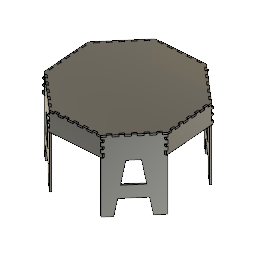
table v11 (Autodesk Fusion 360 design; units mm, degrees)
Autodesk Fusion 360 part; units mm, degrees
note: some values were not read from the file. Chosen so that the rebuilt part matches the saved one: a direction. Set by a fixed rule: which face or edge a step refers to.
sketch "TableTopSide Sketch" plane through (0, 0, 0) normal (0, 0, 1) x (1, 0, 0)
  line L0 (0, 0) -> (123.0551, 378.7517)
  line L1 (123.0551, 378.7517) -> (354.831, 180.8048)
  line L2 (354.831, 180.8048) -> (0, 0)
  dimension "d1" = 45
  dimension "d18" = 304.8
  measures "d1" angle of L0 L2
extrude "Extrude1" add sketch "TableTopSide Sketch" along normal blind 11 makes body 1
sketch "TableTopSideFinger Sketch" plane through (238.9431, 279.7782, 0) normal (0.649432, 0.76042, 0) x (-0.76042, 0.649432, 0)
  line L0 (-152.4, 0) -> (152.4, 0)
  line L1 (152.4, 0) -> (152.4, 11)
  line L2 (152.4, 11) -> (-152.4, 11)
  line L3 (-152.4, 11) -> (-152.4, 0)
  line L4 (-127, 11) -> (-101.6, 11)
  line L5 (-101.6, 11) -> (-101.6, 0)
  line L6 (-101.6, 0) -> (-127, 0)
  line L7 (-127, 0) -> (-127, 11)
  dimension "d23" = 25.4
  dimension "d24" = 25.4
  measures "d23" distance of L3 L7
  measures "d24" distance of L5 L7
extrude "Extrude3" cut sketch "TableTopSideFinger Sketch" against normal blind 11 contours L0 L2 L4 L5 L6 L7 bodies 1
pattern_linear "R-Pattern2" count 5 spacing 57.15 along (-0.76042, 0.649432, 0) of "Extrude3"
pattern_circular "C-Pattern1" count 8 over 360 about axis through (0, 0, 1.75) along (0, 0, 1) of bodies 1 makes body 2 at (-37.6656, 235.7218, 11) makes body 3 at (-193.3141, 140.0469, 11) makes body 4 at (-235.7218, -37.6656, 11) makes body 5 at (-169.0189, -168.5707, 11) makes body 6 at (37.6656, -235.7218, 11) makes body 7 at (193.3141, -140.0469, 11) makes body 8 at (235.7218, 37.6656, 11)
sketch "Leg Sketch" plane through (238.9431, 279.7782, 0) normal (0.649432, 0.76042, 0) x (-0.76042, 0.649432, 0)
  line L0 (-152.4, 11) -> (152.4, 11)
  line L1 (152.4, 11) -> (152.4, -441.7199)
  line L2 (-152.4, -441.7199) -> (-152.4, 11)
  line L3 (152.4, 0) -> (152.4, 11)
  line L4 (-92.9491, -441.7199) -> (-38.655, -133.8025)
  line L5 (-38.655, -133.8025) -> (31.7592, -133.8025)
  line L6 (31.7592, -133.8025) -> (86.0534, -441.7199)
  line L7 (152.4, -441.7199) -> (86.0534, -441.7199)
  line L8 (-92.9491, -441.7199) -> (-152.4, -441.7199)
  line L9 (-75.5345, -342.9565) -> (68.6387, -342.9565)
  line L10 (-62.4641, -268.8305) -> (55.5683, -268.8305)
  dimension "d36" = 100
  dimension "d37" = 100
  measures "d36" angle of L4 L8
  measures "d37" angle of L6 L7
extrude "Extrude4" add sketch "Leg Sketch" against normal blind 11 separate body contours L0 L1 L2 L3 L4 L5 L6 L7 L8 | L4 L6 L9 L10 makes body 9
combine "Combine1" operation cut target body 9 tool bodies 1 keep tools
sketch "SideCover Sketch" plane through (-28.8748, 366.7914, 0) normal (-0.07848, 0.996916, 0) x (-0.996916, -0.07848, 0)
  line L0 (-127, 0) -> (-127, 11)
  line L1 (-127, 11) -> (-152.4, 11)
  line L2 (-152.4, 11) -> (-152.4, 0)
  line L3 (-152.4, 0) -> (-127, 0)
  line L4 (0, 11) -> (0, -115) construction
  line L5 (-163.4, 11) -> (163.4, 11)
  line L6 (163.4, 11) -> (163.4, -111.0995)
  line L7 (163.4, -111.0995) -> (-163.4, -111.0995)
  line L8 (-163.4, -111.0995) -> (-163.4, 11)
  line L9 (12.7, 11) -> (44.45, 11)
  line L10 (152.4, 11) -> (152.4, -33.5866) construction
  line L11 (-152.4, 11) -> (-152.4, -39.2984)
  dimension "d61" = 11
  dimension "d62" = 11
  measures "d61" distance of L8 L11
  measures "d62" distance of L6 L10
extrude "Extrude5" add sketch "SideCover Sketch" against normal blind 11 separate body makes body 10
sketch "SideCoverFinger Sketch" plane through (162.896, 12.8236, 0) normal (0.996916, 0.07848, 0) x (-0.07848, 0.996916, 0)
  line L0 (367.9261, -115) -> (367.9261, 0)
  line L1 (367.9261, 0) -> (355.9261, 0)
  line L2 (355.9261, 0) -> (355.9261, -115)
  line L3 (355.9261, -115) -> (367.9261, -115)
  line L4 (355.9261, -13.4) -> (367.9261, -13.4)
  line L5 (367.9261, -13.4) -> (367.9261, 12)
  line L6 (367.9261, 12) -> (355.9261, 12)
  line L7 (355.9261, 12) -> (355.9261, -13.4)
  line L8 (367.9261, 12) -> (152.4, 12)
  line L9 (367.9261, -111.0995) -> (367.9261, 11)
  line L10 (367.9261, 11) -> (356.9261, 11)
  line L11 (356.9261, 11) -> (356.9261, -111.0995)
  line L12 (356.9261, -111.0995) -> (367.9261, -111.0995)
  dimension "d46" = 25.4
  measures "d46" distance of L4 L6
extrude "Extrude6" cut sketch "SideCoverFinger Sketch" against normal blind 11 contours L0 L1 L4 L5 L9 L11 | L1 L2 L4 L7 L11 | L1 L5 L9 L10 L11 | L1 L5 L6 L7 L8 L10 L11 bodies 10
pattern_linear "R-Pattern3" count 3 spacing 38.1 along (0, 0, -1) of "Extrude6"
extrude "Extrude8" cut 3 faces at (123.3429, 375.0963, -5.2667) (123.6307, 371.441, -34.5667) (123.6307, 371.441, -72.6667) along direction (0.996916, 0.07848, 0) blind 12 start surface through (-191.7708, 353.9677, 11) normal (-0.996916, -0.07848, 0) on bodies 10 bodies 10
combine "Combine3" operation cut target body 9 tool bodies 10 keep tools
revolve "Revolve1" cut 1 faces at (126.0597, 367.9542, -103.933) angle 45 about axis through (134.8845, 368.6489, -64.2) along (0, 0, 1) on bodies 9 bodies 9
pattern_circular "C-Pattern3" count 4 over 360 about axis through (0, 0, 1.75) along (0, 0, 1) of bodies 10 makes body 11 at (-351.8908, -77.9902, -43.0333) makes body 12 at (77.9902, -351.8908, -43.0333) makes body 13 at (351.8908, 77.9902, -43.0333)
combine "Combine4" operation cut target body 9 tool bodies 13 keep tools
combine "Combine5" operation add target body 1 tool bodies 6 3 2 4 5 7 8 keep tools
revolve "Revolve2" cut 1 faces at (343.7225, 181.7504, -103.933) angle 45 about axis through (343.0017, 190.9076, -51.5) along (0, 0, -1) on bodies 9 bodies 9
pattern_circular "C-Pattern5" count 4 over 360 about axis through (0, 0, 1.75) along (0, 0, 1) of bodies 9 makes body 14 at (-360.6193, 144.2864, -298.592) makes body 15 at (-144.2864, -360.6193, -298.592) makes body 16 at (360.6193, -144.2864, -298.592)
sketch "Sketch8" plane through (366.7914, 28.8748, 0) normal (0.996916, 0.07848, 0) x (-0.07848, 0.996916, 0)
  line L0 (718.5635, -1934.0264) -> (737.8781, -1950.5219)
  line L1 (737.8781, -1950.5219) -> (745.0219, -1942.1573)
  line L2 (745.0219, -1942.1573) -> (764.3365, -1958.6529)
  line L3 (764.3365, -1958.6529) -> (757.1928, -1967.0175)
  line L4 (757.1928, -1967.0175) -> (781.3361, -1987.637)
  line L5 (781.3361, -1987.637) -> (788.4799, -1979.2724)
  line L6 (788.4799, -1979.2724) -> (807.7945, -1995.768)
  line L7 (807.7945, -1995.768) -> (800.6508, -2004.1326)
  line L8 (800.6508, -2004.1326) -> (824.7941, -2024.752)
  line L9 (824.7941, -2024.752) -> (831.9378, -2016.3874)
  line L10 (831.9378, -2016.3874) -> (851.2525, -2032.883)
  line L11 (851.2525, -2032.883) -> (844.1087, -2041.2476)
  line L12 (844.1087, -2041.2476) -> (868.2521, -2061.8671)
  line L13 (868.2521, -2061.8671) -> (875.3958, -2053.5025)
  line L14 (875.3958, -2053.5025) -> (894.7105, -2069.998)
  line L15 (894.7105, -2069.998) -> (887.5667, -2078.3627)
  line L16 (887.5667, -2078.3627) -> (911.71, -2098.9821)
  line L17 (911.71, -2098.9821) -> (918.8538, -2090.6175)
  line L18 (918.8538, -2090.6175) -> (938.1684, -2107.1131)
  line L19 (938.1684, -2107.1131) -> (931.0247, -2115.4777)
  line L20 (931.0247, -2115.4777) -> (950.3393, -2131.9733)
  line L21 (950.3393, -2131.9733) -> (975.661, -2129.9799)
  line L22 (975.661, -2129.9799) -> (974.7977, -2119.0138)
  line L23 (974.7977, -2119.0138) -> (1000.1194, -2117.0204)
  line L24 (1000.1194, -2117.0204) -> (1000.9827, -2127.9865)
  line L25 (1000.9827, -2127.9865) -> (1032.6347, -2125.4948)
  line L26 (1032.6347, -2125.4948) -> (1031.7715, -2114.5287)
  line L27 (1031.7715, -2114.5287) -> (1057.0931, -2112.5353)
  line L28 (1057.0931, -2112.5353) -> (1057.9564, -2123.5014)
  line L29 (1057.9564, -2123.5014) -> (1089.6085, -2121.0096)
  line L30 (1089.6085, -2121.0096) -> (1088.7452, -2110.0436)
  line L31 (1088.7452, -2110.0436) -> (1114.0668, -2108.0502)
  line L32 (1114.0668, -2108.0502) -> (1114.9301, -2119.0163)
  line L33 (1114.9301, -2119.0163) -> (1146.5822, -2116.5245)
  line L34 (1146.5822, -2116.5245) -> (1145.7189, -2105.5584)
  line L35 (1145.7189, -2105.5584) -> (1171.0406, -2103.5651)
  line L36 (1171.0406, -2103.5651) -> (1171.9039, -2114.5311)
  line L37 (1171.9039, -2114.5311) -> (1203.5559, -2112.0394)
  line L38 (1203.5559, -2112.0394) -> (1202.6926, -2101.0733)
  line L39 (1202.6926, -2101.0733) -> (1228.0143, -2099.0799)
  line L40 (1228.0143, -2099.0799) -> (1228.8776, -2110.046)
  line L41 (1228.8776, -2110.046) -> (1254.1992, -2108.0526)
  line L42 (1254.1992, -2108.0526) -> (1270.6948, -2088.738)
  line L43 (1270.6948, -2088.738) -> (1262.3302, -2081.5942)
  line L44 (1262.3302, -2081.5942) -> (1278.8258, -2062.2795)
  line L45 (1278.8258, -2062.2795) -> (1287.1904, -2069.4233)
  line L46 (1287.1904, -2069.4233) -> (1307.8099, -2045.28)
  line L47 (1307.8099, -2045.28) -> (1299.4453, -2038.1362)
  line L48 (1299.4453, -2038.1362) -> (1315.9408, -2018.8216)
  line L49 (1315.9408, -2018.8216) -> (1324.3054, -2025.9653)
  line L50 (1324.3054, -2025.9653) -> (1344.9249, -2001.822)
  line L51 (1344.9249, -2001.822) -> (1336.5603, -1994.6782)
  line L52 (1336.5603, -1994.6782) -> (1353.0559, -1975.3636)
  line L53 (1353.0559, -1975.3636) -> (1361.4205, -1982.5073)
  line L54 (1361.4205, -1982.5073) -> (1382.04, -1958.364)
  line L55 (1382.04, -1958.364) -> (1373.6753, -1951.2203)
  line L56 (1373.6753, -1951.2203) -> (1390.1709, -1931.9056)
  line L57 (1390.1709, -1931.9056) -> (1398.5355, -1939.0494)
  line L58 (1398.5355, -1939.0494) -> (1419.155, -1914.906)
  line L59 (1419.155, -1914.906) -> (1410.7904, -1907.7623)
  line L60 (1410.7904, -1907.7623) -> (1427.286, -1888.4476)
  line L61 (1427.286, -1888.4476) -> (1435.6506, -1895.5914)
  line L62 (1435.6506, -1895.5914) -> (1452.1462, -1876.2767)
  line L63 (1452.1462, -1876.2767) -> (1450.1528, -1850.9551)
  line L64 (1450.1528, -1850.9551) -> (1439.1867, -1851.8184)
  line L65 (1439.1867, -1851.8184) -> (1437.1933, -1826.4967)
  line L66 (1437.1933, -1826.4967) -> (1448.1594, -1825.6334)
  line L67 (1448.1594, -1825.6334) -> (1445.6676, -1793.9813)
  line L68 (1445.6676, -1793.9813) -> (1434.7016, -1794.8446)
  line L69 (1434.7016, -1794.8446) -> (1432.7082, -1769.523)
  line L70 (1432.7082, -1769.523) -> (1443.6743, -1768.6597)
  line L71 (1443.6743, -1768.6597) -> (1441.1825, -1737.0076)
  line L72 (1441.1825, -1737.0076) -> (1430.2164, -1737.8709)
  line L73 (1430.2164, -1737.8709) -> (1428.2231, -1712.5492)
  line L74 (1428.2231, -1712.5492) -> (1439.1891, -1711.686)
  line L75 (1439.1891, -1711.686) -> (1436.6974, -1680.0339)
  line L76 (1436.6974, -1680.0339) -> (1425.7313, -1680.8972)
  line L77 (1425.7313, -1680.8972) -> (1423.7379, -1655.5755)
  line L78 (1423.7379, -1655.5755) -> (1434.704, -1654.7122)
  line L79 (1434.704, -1654.7122) -> (1432.2123, -1623.0601)
  line L80 (1432.2123, -1623.0601) -> (1421.2462, -1623.9234)
  line L81 (1421.2462, -1623.9234) -> (1419.2528, -1598.6018)
  line L82 (1419.2528, -1598.6018) -> (1430.2189, -1597.7385)
  line L83 (1430.2189, -1597.7385) -> (1428.2255, -1572.4168)
  line L84 (1428.2255, -1572.4168) -> (1408.9108, -1555.9213)
  line L85 (1408.9108, -1555.9213) -> (1401.7671, -1564.2859)
  line L86 (1401.7671, -1564.2859) -> (1382.4524, -1547.7903)
  line L87 (1382.4524, -1547.7903) -> (1389.5962, -1539.4257)
  line L88 (1389.5962, -1539.4257) -> (1365.4529, -1518.8062)
  line L89 (1365.4529, -1518.8062) -> (1358.3091, -1527.1708)
  line L90 (1358.3091, -1527.1708) -> (1338.9944, -1510.6752)
  line L91 (1338.9944, -1510.6752) -> (1346.1382, -1502.3106)
  line L92 (1346.1382, -1502.3106) -> (1321.9949, -1481.6912)
  line L93 (1321.9949, -1481.6912) -> (1314.8511, -1490.0558)
  line L94 (1314.8511, -1490.0558) -> (1295.5365, -1473.5602)
  line L95 (1295.5365, -1473.5602) -> (1302.6802, -1465.1956)
  line L96 (1302.6802, -1465.1956) -> (1278.5369, -1444.5761)
  line L97 (1278.5369, -1444.5761) -> (1271.3931, -1452.9407)
  line L98 (1271.3931, -1452.9407) -> (1252.0785, -1436.4451)
  line L99 (1252.0785, -1436.4451) -> (1259.2222, -1428.0805)
  line L100 (1259.2222, -1428.0805) -> (1235.0789, -1407.4611)
  line L101 (1235.0789, -1407.4611) -> (1227.9352, -1415.8257)
  line L102 (1227.9352, -1415.8257) -> (1208.6205, -1399.3301)
  line L103 (1208.6205, -1399.3301) -> (1215.7643, -1390.9655)
  line L104 (1215.7643, -1390.9655) -> (1196.4496, -1374.4699)
  line L105 (1196.4496, -1374.4699) -> (1171.128, -1376.4633)
  line L106 (1171.128, -1376.4633) -> (1171.9912, -1387.4294)
  line L107 (1171.9912, -1387.4294) -> (1146.6696, -1389.4228)
  line L108 (1146.6696, -1389.4228) -> (1145.8063, -1378.4567)
  line L109 (1145.8063, -1378.4567) -> (1114.1542, -1380.9484)
  line L110 (1114.1542, -1380.9484) -> (1115.0175, -1391.9145)
  line L111 (1115.0175, -1391.9145) -> (1089.6958, -1393.9079)
  line L112 (1089.6958, -1393.9079) -> (1088.8326, -1382.9418)
  line L113 (1088.8326, -1382.9418) -> (1057.1805, -1385.4336)
  line L114 (1057.1805, -1385.4336) -> (1058.0438, -1396.3996)
  line L115 (1058.0438, -1396.3996) -> (1032.7221, -1398.393)
  line L116 (1032.7221, -1398.393) -> (1031.8588, -1387.4269)
  line L117 (1031.8588, -1387.4269) -> (1000.2068, -1389.9187)
  line L118 (1000.2068, -1389.9187) -> (1001.07, -1400.8848)
  line L119 (1001.07, -1400.8848) -> (975.7484, -1402.8781)
  line L120 (975.7484, -1402.8781) -> (974.8851, -1391.9121)
  line L121 (974.8851, -1391.9121) -> (943.233, -1394.4038)
  line L122 (943.233, -1394.4038) -> (944.0963, -1405.3699)
  line L123 (944.0963, -1405.3699) -> (918.7746, -1407.3633)
  line L124 (918.7746, -1407.3633) -> (917.9114, -1396.3972)
  line L125 (917.9114, -1396.3972) -> (892.5897, -1398.3906)
  line L126 (892.5897, -1398.3906) -> (876.0941, -1417.7052)
  line L127 (876.0941, -1417.7052) -> (884.4587, -1424.849)
  line L128 (884.4587, -1424.849) -> (867.9632, -1444.1637)
  line L129 (867.9632, -1444.1637) -> (859.5986, -1437.0199)
  line L130 (859.5986, -1437.0199) -> (838.9791, -1461.1632)
  line L131 (838.9791, -1461.1632) -> (847.3437, -1468.307)
  line L132 (847.3437, -1468.307) -> (830.8481, -1487.6216)
  line L133 (830.8481, -1487.6216) -> (822.4835, -1480.4779)
  line L134 (822.4835, -1480.4779) -> (801.864, -1504.6212)
  line L135 (801.864, -1504.6212) -> (810.2287, -1511.7649)
  line L136 (810.2287, -1511.7649) -> (793.7331, -1531.0796)
  line L137 (793.7331, -1531.0796) -> (785.3685, -1523.9359)
  line L138 (785.3685, -1523.9359) -> (764.749, -1548.0792)
  line L139 (764.749, -1548.0792) -> (773.1136, -1555.2229)
  line L140 (773.1136, -1555.2229) -> (756.618, -1574.5376)
  line L141 (756.618, -1574.5376) -> (748.2534, -1567.3938)
  line L142 (748.2534, -1567.3938) -> (727.6339, -1591.5371)
  line L143 (727.6339, -1591.5371) -> (735.9986, -1598.6809)
  line L144 (735.9986, -1598.6809) -> (719.503, -1617.9956)
  line L145 (719.503, -1617.9956) -> (711.1384, -1610.8518)
  line L146 (711.1384, -1610.8518) -> (694.6428, -1630.1665)
  line L147 (694.6428, -1630.1665) -> (696.6362, -1655.4881)
  line L148 (696.6362, -1655.4881) -> (707.6022, -1654.6248)
  line L149 (707.6022, -1654.6248) -> (709.5956, -1679.9465)
  line L150 (709.5956, -1679.9465) -> (698.6296, -1680.8098)
  line L151 (698.6296, -1680.8098) -> (701.1213, -1712.4619)
  line L152 (701.1213, -1712.4619) -> (712.0874, -1711.5986)
  line L153 (712.0874, -1711.5986) -> (714.0808, -1736.9202)
  line L154 (714.0808, -1736.9202) -> (703.1147, -1737.7835)
  line L155 (703.1147, -1737.7835) -> (705.6064, -1769.4356)
  line L156 (705.6064, -1769.4356) -> (716.5725, -1768.5723)
  line L157 (716.5725, -1768.5723) -> (718.5659, -1793.894)
  line L158 (718.5659, -1793.894) -> (707.5998, -1794.7572)
  line L159 (707.5998, -1794.7572) -> (710.0916, -1826.4093)
  line L160 (710.0916, -1826.4093) -> (721.0576, -1825.546)
  line L161 (721.0576, -1825.546) -> (723.051, -1850.8677)
  line L162 (723.051, -1850.8677) -> (712.0849, -1851.731)
  line L163 (712.0849, -1851.731) -> (714.5767, -1883.383)
  line L164 (714.5767, -1883.383) -> (725.5428, -1882.5198)
  line L165 (725.5428, -1882.5198) -> (727.5361, -1907.8414)
  line L166 (727.5361, -1907.8414) -> (716.5701, -1908.7047)
  line L167 (716.5701, -1908.7047) -> (718.5635, -1934.0264)
  line L168 (163.4, -51.5) -> (151.4, -51.5)
  line L169 (151.4, -51.5) -> (151.4, -26.1)
  line L170 (151.4, -26.1) -> (163.4, -26.1)
  line L171 (163.4, -26.1) -> (163.4, -13.4)
  line L172 (163.4, -13.4) -> (151.4, -13.4)
  line L173 (151.4, -13.4) -> (151.4, 11)
  line L174 (151.4, 11) -> (-152.4, 11)
  line L175 (-152.4, 11) -> (-152.4, -13.4)
  line L176 (-152.4, -13.4) -> (-163.4, -13.4)
  line L177 (-163.4, -13.4) -> (-163.4, -26.1)
  line L178 (-163.4, -26.1) -> (-152.4, -26.1)
  line L179 (-152.4, -26.1) -> (-152.4, -51.5)
  line L180 (-152.4, -51.5) -> (-163.4, -51.5)
  line L181 (-163.4, -51.5) -> (-163.4, -64.2)
  line L182 (-163.4, -64.2) -> (-152.4, -64.2)
  line L183 (-152.4, -64.2) -> (-152.4, -89.6)
  line L184 (-152.4, -89.6) -> (-163.4, -89.6)
  line L185 (-163.4, -89.6) -> (-163.4, -111.0995)
  line L186 (-163.4, -111.0995) -> (163.4, -111.0995)
  line L187 (163.4, -111.0995) -> (163.4, -89.6)
  line L188 (163.4, -89.6) -> (151.4, -89.6)
  line L189 (151.4, -89.6) -> (151.4, -64.2)
  line L190 (151.4, -64.2) -> (163.4, -64.2)
  line L191 (163.4, -64.2) -> (163.4, -51.5)
combine "Combine7" operation cut target body 10 tool bodies 2 keep tools
extrude "Extrude10" cut 2 faces at (-177.9874, 346.8896, 11) (122.1166, 371.3218, 11) along direction (0, 0, -1) blind 11 on bodies 10 bodies 10
combine "Combine8" operation cut target body 13 tool bodies 8 keep tools
combine "Combine9" operation cut target body 12 tool bodies 6 keep tools
combine "Combine10" operation cut target body 11 tool bodies 4 keep tools
extrude "Extrude11" cut 2 faces at (346.8896, 177.9874, 11) (371.3218, -122.1166, 11) along direction (0, 0, -1) blind 11 on bodies 13 bodies 13
extrude "Extrude12" cut 2 faces at (-122.1166, -371.3218, 11) (177.9874, -346.8896, 11) along direction (0, 0, -1) blind 11 on bodies 12 bodies 12
extrude "Extrude13" cut 2 faces at (-371.3218, 122.1166, 11) (-346.8896, -177.9874, 11) along direction (0, 0, -1) blind 11 on bodies 11 bodies 11
extrude "Extrude14" cut 1 faces at (180.0508, -353.7488, 11) along direction (0, 0, -1) blind 11 on bodies 16 bodies 16
extrude "Extrude15" cut 1 faces at (-353.7488, -180.0508, 11) along direction (0, 0, -1) blind 11 on bodies 15 bodies 15
extrude "Extrude16" cut 1 faces at (-180.0508, 353.7488, 11) along direction (0, 0, -1) blind 11 on bodies 14 bodies 14
extrude "Extrude17" cut 1 faces at (353.7488, 180.0508, 11) along direction (0, 0, -1) blind 11 on bodies 9 bodies 9
copy_body "CopyPasteBodies1" bodies 10 makes body 17 in component "SideCover"
sketch "Sketch1" plane through (-28.0115, 355.8253, 0) normal (0.07848, -0.996916, 0) x (0.996916, 0.07848, 0) in component "SideCover"
  line L0 (-127, 0) -> (-151.4, 0)
  line L1 (-151.4, 0) -> (-151.4, -13.4)
  line L2 (-151.4, -13.4) -> (-163.4, -13.4)
  line L3 (-163.4, -13.4) -> (-163.4, -26.1)
  line L4 (-163.4, -26.1) -> (-151.4, -26.1)
  line L5 (-151.4, -26.1) -> (-151.4, -51.5)
  line L6 (-151.4, -51.5) -> (-163.4, -51.5)
  line L7 (-163.4, -51.5) -> (-163.4, -64.2)
  line L8 (-163.4, -64.2) -> (-151.4, -64.2)
  line L9 (-151.4, -64.2) -> (-151.4, -89.6)
  line L10 (-151.4, -89.6) -> (-163.4, -89.6)
  line L11 (-163.4, -89.6) -> (-163.4, -111.0995)
  line L12 (-163.4, -111.0995) -> (163.4, -111.0995)
  line L13 (163.4, -111.0995) -> (163.4, -89.6)
  line L14 (163.4, -89.6) -> (152.4, -89.6)
  line L15 (152.4, -89.6) -> (152.4, -64.2)
  line L16 (152.4, -64.2) -> (163.4, -64.2)
  line L17 (163.4, -64.2) -> (163.4, -51.5)
  line L18 (163.4, -51.5) -> (152.4, -51.5)
  line L19 (152.4, -51.5) -> (152.4, -26.1)
  line L20 (152.4, -26.1) -> (163.4, -26.1)
  line L21 (163.4, -26.1) -> (163.4, -13.4)
  line L22 (163.4, -13.4) -> (152.4, -13.4)
  line L23 (152.4, -13.4) -> (152.4, 0)
  line L24 (152.4, 0) -> (127, 0)
  line L25 (127, 0) -> (127, 11)
  line L26 (127, 11) -> (101.6, 11)
  line L27 (101.6, 11) -> (101.6, 0)
  line L28 (101.6, 0) -> (69.85, 0)
  line L29 (69.85, 0) -> (69.85, 11)
  line L30 (69.85, 11) -> (44.45, 11)
  line L31 (44.45, 11) -> (44.45, 0)
  line L32 (44.45, 0) -> (12.7, 0)
  line L33 (12.7, 0) -> (12.7, 11)
  line L34 (12.7, 11) -> (-12.7, 11)
  line L35 (-12.7, 11) -> (-12.7, 0)
  line L36 (-12.7, 0) -> (-44.45, 0)
  line L37 (-44.45, 0) -> (-44.45, 11)
  line L38 (-44.45, 11) -> (-69.85, 11)
  line L39 (-69.85, 11) -> (-69.85, 0)
  line L40 (-69.85, 0) -> (-101.6, 0)
  line L41 (-101.6, 0) -> (-101.6, 11)
  line L42 (-101.6, 11) -> (-127, 11)
  line L43 (-127, 11) -> (-127, 0)
copy_body "Body->Comp1" bodies 1 removing the originals makes body 18 in component "TableTop"
copy_body "Body->Comp2" bodies 9 removing the originals makes body 19 in component "LegExtrude"
copy_body "Body->Comp3" bodies 14 removing the originals makes body 20 in component "LegExtrude (1)"
copy_body "Body->Comp4" bodies 15 removing the originals makes body 21 in component "LegExtrude (2)"
copy_body "Body->Comp5" bodies 16 removing the originals makes body 22 in component "LegExtrude (3)"
copy_body "Body->Comp6" bodies 10 removing the originals makes body 23 in component "SideCoverExtrude"
copy_body "Body->Comp7" bodies 11 removing the originals makes body 24 in component "SideCoverExtrude (1)"
copy_body "Body->Comp8" bodies 12 removing the originals makes body 25 in component "SideCoverExtrude (2)"
copy_body "Body->Comp9" bodies 13 removing the originals makes body 26 in component "SideCoverExtrude (3)"
component "SideCover" placed x (1, 0, 0) y (0, 1, 0) z (0, 0, 1) at (0, 0, 0)
component "TableTop" placed x (1, 0, 0) y (0, 1, 0) z (0, 0, 1) at (0, 0, 0)
component "LegExtrude" placed x (1, 0, 0) y (0, 1, 0) z (0, 0, 1) at (0, 0, 0)
component "LegExtrude (1)" placed x (1, 0, 0) y (0, 1, 0) z (0, 0, 1) at (0, 0, 0)
component "LegExtrude (2)" placed x (1, 0, 0) y (0, 1, 0) z (0, 0, 1) at (0, 0, 0)
component "LegExtrude (3)" placed x (1, 0, 0) y (0, 1, 0) z (0, 0, 1) at (0, 0, 0)
component "SideCoverExtrude" placed x (1, 0, 0) y (0, 1, 0) z (0, 0, 1) at (0, 0, 0)
component "SideCoverExtrude (1)" placed x (1, 0, 0) y (0, 1, 0) z (0, 0, 1) at (0, 0, 0)
component "SideCoverExtrude (2)" placed x (1, 0, 0) y (0, 1, 0) z (0, 0, 1) at (0, 0, 0)
component "SideCoverExtrude (3)" placed x (1, 0, 0) y (0, 1, 0) z (0, 0, 1) at (0, 0, 0)
hidden bodies 3 4 5 6 7 8
equation "d1 = ( 360 / sides ) * 1 deg"
equation "materialThickness = 11 mm"
equation "fingerJointSize = 1 in"
equation "d5 = materialThickness"
equation "d18 = tableSide"
equation "tableSide = 12 * fingerJointSize"
equation "d23 = fingerJointSize"
equation "d24 = fingerJointSize"
equation "d26 = -materialThickness"
equation "nFingerSide = ( tableSide / fingerJointSize ) / 2"
equation "d29 = nFingerSide - 1"
equation "d31 = tableSide - ( 3 * fingerJointSize )"
equation "sides = 8"
equation "d34 = sides"
equation "d39 = -materialThickness"
equation "d44 = -materialThickness"
equation "d46 = fingerJointSize"
equation "sideCoverHeight = 5 * fingerJointSize"
equation "d51 = -materialThickness"
equation "d53 = floor(sideCoverHeight / fingerJointSize) - 2"
equation "d55 = sideCoverHeight - 2 * fingerJointSize"
equation "d61 = materialThickness"
equation "d62 = materialThickness"
equation "d66 = ( -360 / sides ) * 1 deg"
equation "d70 = sides / 2"
equation "d74 = ( -360 / sides ) * 1 deg"
equation "d75 = sides / 2"
equation "d77 = -materialThickness"
equation "d79 = -materialThickness"
equation "d81 = -materialThickness"
equation "d83 = -materialThickness"
equation "d85 = -materialThickness"
equation "d87 = -materialThickness"
equation "d89 = -materialThickness"
equation "d91 = -materialThickness"
named bodies: "TableSide Extrude", "LegExtrude", "SideCoverExtrude", "SideCoverExtrude (1)", "SideCoverExtrude (2)", "SideCoverExtrude (3)", "LegExtrude (1)", "LegExtrude (2)", "LegExtrude (3)"
